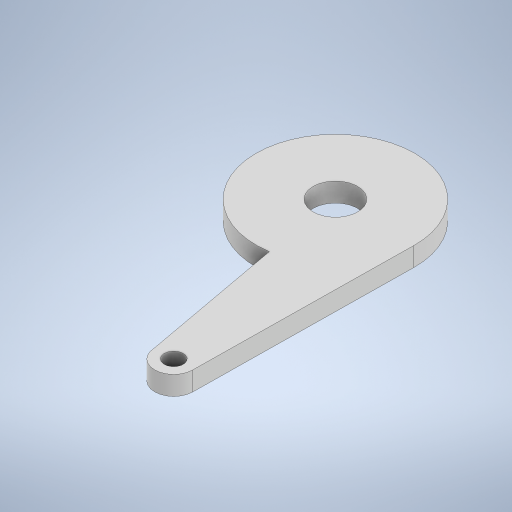
# Autodesk Inventor part: Pinza_pieza4
Saved by Autodesk Inventor 2023 (Build 270158000, 158)
## iProperties
Created: 2024-09-28
Part Number: Pinza_pieza4
Material: Genérico
Document SubType Name: Sheet Metal
Designer: sebas
Density: 1 g/cm^3
Sheet Metal Rule: Por defecto_mm
Appearance: Valor por defecto
Author: sebas
Autodesk Inventor part; units mm, degrees
ref_plane "YZ Plane" through (0, 0, 0) normal (1, 0, 0) x (0, 1, 0)
ref_plane "XZ Plane" through (0, 0, 0) normal (0, 1, 0) x (-1, 0, 0)
ref_plane "XY Plane" through (0, 0, 0) normal (0, 0, 1) x (1, 0, 0)
sketch "Boceto1" plane through (0, 0, 0) normal (0, 1, 0) x (-1, 0, 0)
  line L0 (0, -17.2515) -> (0, 17.2515) construction
  line L1 (-2.9997, 17.2904) -> (-3.4466, -17.089)
  arc A0 (2.999, 17.3273) -> (-2.9997, 17.2904) centre (0, 17.2515) ccw
  circle A1 centre (0, 17.2515) radius 1.5
  arc A2 (-3.4466, -17.089) -> (7.0947, -4.9057) centre (9.0523, -17.2515) ccw
  line L2 (0, -17.2515) -> (12.8049, -17.2515) construction
  line L3 (2.999, 17.3273) -> (7.0947, -4.9057)
  circle A3 centre (9.0523, -17.2515) radius 3.5
  point P0 (0, 0)
  point P1 (9.3192, -29.7486)
  point P2 (-0.0184, 20.2514)
  dimension "d0" = 6
  dimension "d1" = 3
  dimension "d3" = 12.5
  dimension "d4" = 50
  dimension "d5" = 7
  constraints: 11 end point, 6 point on circle, 4 centre point, 3 coincident, 2 tangent, 1 horizontal, 1 midpoint, 1 point on line, 1 vertical
  measures "d0" diameter of A0
  measures "d1" diameter of A1
  measures "d3" radius of A2
  measures "d4" vertical distance of point (-0.018, 20.251) point (9.319, -29.749)
  measures "d5" diameter of A3
extrude "Extrusión1" add sketch "Boceto1" along normal mid plane 3
equation "\"Radio_pliegue\" = Grosor"
equation "\"Anchura_desahogo_plegado\" = Grosor"
equation "\"Profundidad_desahogo_plegado\" = 0.5 * Grosor"
equation "\"Tamaño_destalonado\" = 4 * Grosor"
equation "\"Remanente_mínimo\" = 2 * Grosor"
equation "\"Radiodetransición\" = Radio_pliegue"
equation "\"Tamaño_de_radio_de_Jacobi\" = Radio_pliegue"
equation "\"TamañoSeparación\" = Grosor"
equation "\"Grosor\" = 0.5"
